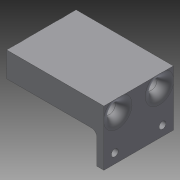
# Autodesk Inventor part: tubing_alignment_arm[3]
Saved by Autodesk Inventor 2015 (Build 190159000, 159)
## iProperties
Created: 2017-04-13
Part Number: tubing_alignment_arm[3]
Material: Generic
Document SubType Name: Modeling
Designer: Guy
Density: 1 g/cm^3
Appearance: Default
Author: Guy
Autodesk Inventor part; units mm, degrees
ref_plane "YZ Plane" through (0, 0, 0) normal (1, 0, 0) x (0, 1, 0)
ref_plane "XZ Plane" through (0, 0, 0) normal (0, 1, 0) x (-1, 0, 0)
ref_plane "XY Plane" through (0, 0, 0) normal (0, 0, 1) x (1, 0, 0)
sketch "Sketch1" plane through (0, 0, 0) normal (0, 0, 1) x (1, 0, 0)
  line L0 (0, 0) -> (50, 0)
  line L1 (50, 0) -> (50, 40)
  line L2 (50, 40) -> (0, 40)
  line L3 (0, 40) -> (0, 0)
  dimension "d0" = 50
  dimension "d1" = 40
  constraints: 8 end point, 2 parallel, 1 horizontal, 1 perpendicular
  measures "d0" distance of L0.start L0.end
  measures "d1" distance of L2.end L0.start
extrude "Extrusion1" add sketch "Sketch1" along normal blind 70
sketch "Sketch2" plane through (50, 0, 0) normal (1, 0, 0) x (0, 0, -1)
  line L0 (0, 0) -> (0, 40) projected
  line L1 (0, 40) -> (-70, 40) projected
  line L2 (-70, 0) -> (-70, 40) projected
  line L3 (0, 0) -> (-70, 0) projected
  line L4 (-70, 0) -> (-5, 0)
  line L5 (-5, 0) -> (-5, 22)
  line L6 (-5, 22) -> (-70, 22)
  line L7 (-70, 22) -> (-70, 0)
  point P0 (0, 0)
  dimension "d5" = 5
  dimension "d6" = 18
  constraints: 8 end point, 2 parallel, 1 horizontal, 1 perpendicular
  measures "d5" distance between parallel lines of L0 L5
  measures "d6" distance between parallel lines of L6 L1
extrude "Extrusion2" cut sketch "Sketch2" against normal up to next contours L3 L2 L6 L5
sketch "Sketch3" plane through (0, 0, 70) normal (0, 0, 1) x (1, 0, 0)
  line L0 (0, 22) -> (50, 22) projected
  line L1 (50, 22) -> (50, 40) projected
  line L2 (50, 40) -> (0, 40) projected
  line L3 (0, 40) -> (0, 22) projected
  circle A0 centre (10, 31) radius 4.25
  circle A1 centre (40, 31) radius 4.25
  point P0 (0, 0)
  dimension "d9" = 8.5
  dimension "d10" = 8.5
  dimension "d11" = 30
  dimension "d12" = 50
  dimension "d13" = 10
  dimension "d14" = 18
  dimension "d15" = 9
  dimension "d16" = 9
  constraints: 2 centre point
  measures "d9" diameter of A1
  measures "d10" diameter of A0
  measures "d11" distance of A1.centre A0.centre
  measures "d12" distance of L1.end L2.end
  measures "d13" distance from line of L3 A0.centre
  measures "d14" distance between parallel lines of L0 L2
  measures "d15" distance from line of A0.centre L2
  measures "d16" distance from line of A1.centre L2
extrude "Extrusion3" cut sketch "Sketch3" against normal up to next contours A0 | A1
fillet "Fillet1" radius 4 1 edges at (25, 22, 5)
sketch "Sketch4" plane through (0, 0, 0) normal (0, 0, -1) x (-1, 0, 0)
  circle A0 centre (-10, 31) radius 4.25 projected
  circle A1 centre (-40, 31) radius 4.25 projected
  line L0 (0, 0) -> (-50, 0) projected
  line L1 (0, 40) -> (0, 0) projected
  line L2 (-50, 40) -> (0, 40) projected
  line L3 (-50, 0) -> (-50, 40) projected
  circle A2 centre (-42.175, 7) radius 2.5
  circle A3 centre (-7.825, 7) radius 2.5
  dimension "d20" = 50
  dimension "d21" = 5
  dimension "d22" = 5
  dimension "d23" = 34.35
  dimension "d24" = 7.825
  dimension "d25" = 7
  dimension "d26" = 7
  constraints: 2 centre point
  measures "d20" distance of L0.start L0.end
  measures "d21" diameter of A3
  measures "d22" diameter of A2
  measures "d23" distance of A3.centre A2.centre
  measures "d24" distance from line of L3 A2.centre
  measures "d25" distance from line of L0 A3.centre
  measures "d26" distance from line of L0 A2.centre
extrude "Extrusion4" cut sketch "Sketch4" against normal up to next contours A2 | A3
fillet "Fillet2" radius 6 4 edges at (35.75, 31, 0) (5.75, 31, 0) (35.75, 31, 70) (5.75, 31, 70)
equation "\"d9\" = d10"
equation "\"d13\" = -0.5 * d11 + 0.5 * d12"
equation "\"d15\" = 0.5 * d14"
equation "\"d16\" = d15"
equation "\"d24\" = -0.5 * d23 + 0.5 * d20"
equation "\"d26\" = d25"
body "Solid1"
